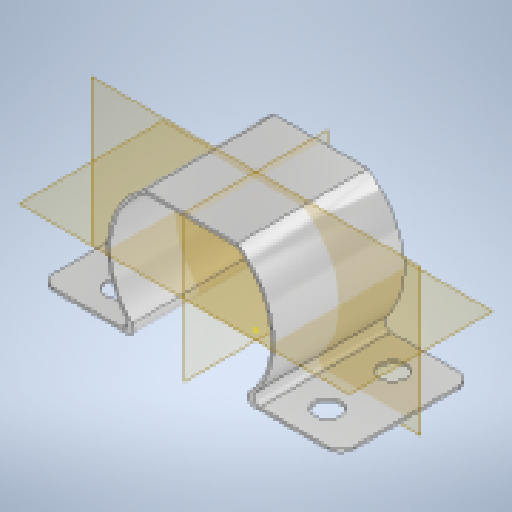
# Autodesk Inventor part: chapa_motor_001
Saved by Autodesk Inventor 2026 (Build 300175000, 175)
## iProperties
Created: 2025-11-27
Part Number: chapa_motor_001
Material: Steel
Document SubType Name: Modeling
Designer: Carlos Dias
Density: 7.85 g/cm^3
Appearance: Aluminum - Dark
Author: Carlos Dias
Autodesk Inventor part; units mm, degrees
sketch "Sketch1" plane through (0, 0, 0) normal (0, 0, 1) x (1, 0, 0)
  line L0 (-6, 5) -> (6, 5) construction
  line L1 (6, 5) -> (6, -5) construction
  line L2 (6, -5) -> (-6, -5) construction
  line L3 (-6, -5) -> (-6, 5) construction
  line L4 (-6, 5) -> (6, -5) construction
  line L5 (6, 5) -> (-6, -5) construction
  line L6 (-3.5, 5) -> (3.5, 5)
  line L7 (-3.5, -5) -> (3.5, -5) construction
  arc A0 (-3.5, 5) -> (-3.5, -5) centre (-0.1834, 0) ccw
  arc A1 (3.5, -5) -> (3.5, 5) centre (0.1834, 0) ccw
  line L8 (-11.5, -5) -> (-3.5, -5)
  line L9 (3.5, -5) -> (11.5, -5)
  line L10 (-11.5, -4.8) -> (-4.1077, -4.8)
  arc A2 (-3.5598, 5.2) -> (-4.1077, -4.8) centre (-0.1834, 0) ccw
  line L11 (-3.5598, 5.2) -> (3.5598, 5.2)
  arc A3 (4.1077, -4.8) -> (3.5598, 5.2) centre (0.1834, 0) ccw
  line L12 (4.1077, -4.8) -> (11.5, -4.8)
  line L13 (11.5, -4.8) -> (11.5, -5)
  line L14 (-11.5, -4.8) -> (-11.5, -5)
  point P0 (0, 0)
  point P1 (0, 0)
  point P2 (0, 5)
  point P3 (0, 5)
  point P4 (0, -5)
  point P5 (0, -5)
  dimension "d0" = 10
  dimension "d1" = 12
  dimension "d2" = 7
  dimension "d3" = 6
  dimension "d4" = 6
  dimension "d5" = 8
  dimension "d6" = 0.2
  dimension "d11" = 7
  constraints: 30 end point, 8 midpoint, 8 point on circle, 5 horizontal, 4 centre point, 2 parallel, 2 vertical, 2 vertical alignment, 1 coincident, 1 collinear, 1 perpendicular, 4 other
  measures "d0" distance between parallel lines of L2 L0
  measures "d1" distance between parallel lines of L3 L1
  measures "d2" distance of L6.start L6.end
  measures "d3" radius of A0
  measures "d4" radius of A1
  measures "d5" distance of L7.start L8.start
  measures "d6" distance between parallel lines of L8 L10
  measures "d11" distance of L7.start L7.end
extrude "Extrusion1" add sketch "Sketch1" along normal mid plane 10
fillet "Fillet1" radius 1 4 edges at (-11.5, -4.9, -5) (-11.5, -4.9, 5) (11.5, -4.9, 5) (11.5, -4.9, -5)
sketch "Sketch2" plane through (4.1077, -4.8, 5) normal (0, 1, 0) x (1, 0, 0)
  point P0 (-4.1077, 5)
fillet "Fillet3" radius 0.5 4 edges at (4.1077, -4.8, 0) (3.5, -5, 0) (-3.5, -5, 0) (-4.1077, -4.8, 0)
sketch "Sketch3" plane through (11.5, -4.8, 4) normal (0, 1, 0) x (1, 0, 0)
  circle A0 centre (-3.5, 1.5) radius 1 projected
  circle A1 centre (-3.5, 6.5) radius 1 projected
  circle A2 centre (-19.5, 6.5) radius 1 projected
  circle A3 centre (-19.5, 1.5) radius 1 projected
  point P0 (-11.5, 4)
extrude "Extrusion2" cut sketch "Sketch3" against normal through all
body "Solid1"
